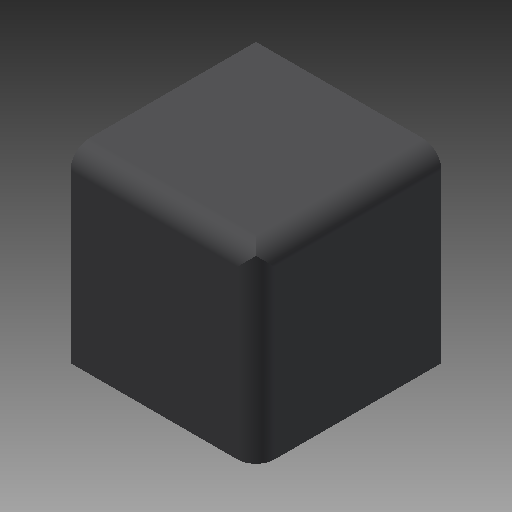
# Autodesk Inventor part: May Tec 1.48.14410_Corner piece set cubic PA
Saved by Autodesk Inventor 2018 (Build 220112000, 112)
## iProperties
Category: PARTsolutions
Company: MAYTEC
Created: 2012-11-13
Part Number: May Tec 1.48.14410_Corner piece set cubic PA
Catalog Web Link: www.cadenas.de
Description: 1.48.144xx-Corner pieces
Vendor: MAYTEC
Document SubType Name: Modeling
Designer: PARTuser1
Manufacturer: MAYTEC
Density: 1 g/cm^3
Material: Generic
Appearance: RGB(175.94999939203154,175.94999939203154,175.94999939203154)
PSOL_IDENT_0: {\\10.0.0.242\data_v9\23d-libs\maytec\maytec_3d\einbauzubehoer\eckstuecke\1.48.144xx.prj},234 {VTYP=
PSOL_IDENT_1: 3D},{NB=May Tec 1.48.14410_Corner piece set cubic PA},{LINA=May Tec 1.48.14410_Corner piece set cubi
PSOL_IDENT_2: c PA},{NN=1.48.144xx},{DATE=14.09.2010 08:34:28},{GEOMDATE=28.01.2010 00:00:00},{VERSION=},{LINEID=1
PSOL_IDENT_3: 0},{LINESUBID=-1},{WBVAR=}  {NB=May Tec 1.48.14410_Corner piece set cubic PA},{LINA=May Tec 1.48.144
PSOL_IDENT_4: 10_Corner piece set cubic PA},{KT=DUMMY},{PARTNR=1.48.14410},{DESCRIPTION=Eckstueck-Satz Quadrat PA}
PSOL_IDENT_5: ,{TYP=1},{XTRANS=Corner piece set cubic PA}
CNS_NT: Corner pieces
CNS_NB: May Tec 1.48.14410_Corner piece set cubic PA
CNS_NBSYN: May Tec $PARTNR._$XTRANS.
CNS_LINA: May Tec 1.48.14410_Corner piece set cubic PA
CNS_PARTNR: 1.48.14410
CNS_DESCRIPTION: Corner piece set cubic PA
CNS_TYP: 1
CNS_XTRANS: Corner piece set cubic PA
SUPPLIER: MAYTEC
ARTICLENO: May Tec 1.48.14410_Corner piece set cubic PA
BOMINFO: May Tec 1.48.14410_Corner piece set cubic PA
CREATOR: CADENAS GmbH
Title: May Tec 1.48.14410_Corner piece set cubic PA
Author: Cadenas PARTsolutions
Comments: Corner pieces
Autodesk Inventor part; units mm, degrees
sketch "Sketch_1" plane through (0, 0, 0) normal (0, 0, 1) x (1, 0, 0)
  line L0 (0, 0) -> (37, 0)
  line L1 (37, 0) -> (37, 5)
  line L2 (37, 5) -> (34.4991, 13.372)
  line L3 (34.4991, 13.372) -> (27.5772, 20.294)
  line L4 (27.5772, 20.294) -> (27.5772, 21.9203)
  line L5 (27.5772, 21.9203) -> (21.9203, 27.5772)
  line L6 (21.9203, 27.5772) -> (20.294, 27.5772)
  line L7 (20.294, 27.5772) -> (13.372, 34.4991)
  line L8 (13.372, 34.4991) -> (5, 37)
  line L9 (5, 37) -> (0, 37)
  line L10 (0, 37) -> (0, 0)
  circle A0 centre (19.852, 19.852) radius 4.425
  constraints: 22 end point, 1 centre point
extrude "Extrusion1" add sketch "Sketch_1" along normal blind 5
sketch "Sketch_2" plane through (0, 0, 0) normal (1, 0, 0) x (0, 1, 0)
  line L0 (0, 37) -> (0, 0)
  line L1 (0, 0) -> (37, 0)
  line L2 (37, 0) -> (37, 5)
  line L3 (37, 5) -> (34.4991, 13.372)
  line L4 (34.4991, 13.372) -> (27.5772, 20.294)
  line L5 (27.5772, 20.294) -> (27.5772, 21.9203)
  line L6 (27.5772, 21.9203) -> (21.9203, 27.5772)
  line L7 (21.9203, 27.5772) -> (20.294, 27.5772)
  line L8 (20.294, 27.5772) -> (13.372, 34.4991)
  line L9 (13.372, 34.4991) -> (5, 37)
  line L10 (5, 37) -> (0, 37)
  circle A0 centre (19.852, 19.852) radius 4.425
  constraints: 22 end point, 1 centre point
sketch "Sketch_3" plane through (0, 0, 0) normal (0, 1, 0) x (-1, 0, 0)
  line L0 (0, 37) -> (-5, 37)
  line L1 (-5, 37) -> (-13.372, 34.4991)
  line L2 (-13.372, 34.4991) -> (-20.294, 27.5772)
  line L3 (-20.294, 27.5772) -> (-21.9203, 27.5772)
  line L4 (-21.9203, 27.5772) -> (-27.5772, 21.9203)
  line L5 (-27.5772, 21.9203) -> (-27.5772, 20.294)
  line L6 (-27.5772, 20.294) -> (-34.4991, 13.372)
  line L7 (-34.4991, 13.372) -> (-37, 5)
  line L8 (-37, 5) -> (-37, 0)
  line L9 (-37, 0) -> (0, 0)
  line L10 (0, 0) -> (0, 37)
  circle A0 centre (-19.852, 19.852) radius 4.425
  constraints: 22 end point, 1 centre point
extrude "Extrusion2" add sketch "Sketch_3" along normal blind 5
extrude "Extrusion3" add sketch "Sketch_2" along normal blind 5
sketch "Sketch_4" plane through (0, 0, 0) normal (0, 0, 1) x (1, 0, 0)
  line L0 (2.5, 23.85) -> (2.5, 16.1)
  line L1 (2.5, 16.1) -> (4.35, 16.1)
  line L2 (4.35, 16.1) -> (4.35, 23.85)
  line L3 (4.35, 23.85) -> (2.5, 23.85)
  constraints: 8 end point
extrude "Extrusion4" add sketch "Sketch_4" against normal blind 4 draft -5
sketch "Sketch_5" plane through (0, 0, 0) normal (0, 0, 1) x (1, 0, 0)
  line L0 (16.1, 4.35) -> (16.1, 2.5)
  line L1 (16.1, 2.5) -> (23.85, 2.5)
  line L2 (23.85, 2.5) -> (23.85, 4.35)
  line L3 (23.85, 4.35) -> (16.1, 4.35)
  constraints: 8 end point
extrude "Extrusion5" add sketch "Sketch_5" against normal blind 4 draft -5
sketch "Sketch_6" plane through (0, 0, 0) normal (0, 0, 1) x (1, 0, 0)
  circle A0 centre (5.75, 12.975) radius 1
  constraints: 1 centre point
extrude "Extrusion6" add sketch "Sketch_6" against normal blind 4 draft -5
sketch "Sketch_7" plane through (0, 0, 0) normal (0, 0, 1) x (1, 0, 0)
  circle A0 centre (5.75, 26.975) radius 1
  constraints: 1 centre point
extrude "Extrusion7" add sketch "Sketch_7" against normal blind 4 draft -5
sketch "Sketch_8" plane through (0, 0, 0) normal (0, 0, 1) x (1, 0, 0)
  circle A0 centre (26.975, 5.75) radius 1
  constraints: 1 centre point
extrude "Extrusion8" add sketch "Sketch_8" against normal blind 4 draft -5
sketch "Sketch_9" plane through (0, 0, 0) normal (0, 0, 1) x (1, 0, 0)
  circle A0 centre (12.975, 5.75) radius 1
  constraints: 1 centre point
extrude "Extrusion9" add sketch "Sketch_9" against normal blind 4 draft -5
sketch "Sketch_10" plane through (0, 0, 0) normal (0, 1, 0) x (-1, 0, 0)
  line L0 (-2, 2) -> (-2, 8)
  line L1 (-2, 8) -> (-8, 8)
  line L2 (-8, 8) -> (-8, 2)
  line L3 (-8, 2) -> (-2, 2)
  constraints: 8 end point
extrude "Extrusion10" cut sketch "Sketch_10" along normal blind 8.5
sketch "Sketch_11" plane through (0, 0, 0) normal (0.7071068, 0, -0.7071068) x (-0.7071068, 0, -0.7071068)
  line L0 (-2, 0) -> (0, 0)
  line L1 (0, 0) -> (0, 2)
  line L2 (0, 2) -> (-2, 0)
  constraints: 6 end point
extrude "Extrusion11" cut sketch "Sketch_11" along normal mid plane 6
sketch "Sketch_12" plane through (0, 0, 0) normal (1, 0, 0) x (0, 1, 0)
  line L0 (23.85, 4.35) -> (16.1, 4.35)
  line L1 (16.1, 4.35) -> (16.1, 2.5)
  line L2 (16.1, 2.5) -> (23.85, 2.5)
  line L3 (23.85, 2.5) -> (23.85, 4.35)
  constraints: 8 end point
sketch "Sketch_13" plane through (0, 0, 0) normal (1, 0, 0) x (0, 1, 0)
  circle A0 centre (12.975, 5.75) radius 1
  constraints: 1 centre point
sketch "Sketch_14" plane through (0, 0, 0) normal (1, 0, 0) x (0, 1, 0)
  circle A0 centre (26.975, 5.75) radius 1
  constraints: 1 centre point
extrude "Extrusion12" add sketch "Sketch_14" against normal blind 4 draft -5
sketch "Sketch_15" plane through (0, 0, 0) normal (1, 0, 0) x (0, 1, 0)
  circle A0 centre (5.75, 12.975) radius 1
  constraints: 1 centre point
extrude "Extrusion13" add sketch "Sketch_15" against normal blind 4 draft -5
sketch "Sketch_16" plane through (0, 0, 0) normal (1, 0, 0) x (0, 1, 0)
  line L0 (4.35, 23.85) -> (2.5, 23.85)
  line L1 (2.5, 23.85) -> (2.5, 16.1)
  line L2 (2.5, 16.1) -> (4.35, 16.1)
  line L3 (4.35, 16.1) -> (4.35, 23.85)
  constraints: 8 end point
extrude "Extrusion14" add sketch "Sketch_16" against normal blind 4 draft -5
sketch "Sketch_17" plane through (0, 0, 0) normal (1, 0, 0) x (0, 1, 0)
  circle A0 centre (5.75, 26.975) radius 1
  constraints: 1 centre point
extrude "Extrusion15" add sketch "Sketch_17" against normal blind 4 draft -5
sketch "Sketch_18" plane through (0, 0, 0) normal (0, 1, 0) x (-1, 0, 0)
  line L0 (-16.1, 4.35) -> (-23.85, 4.35)
  line L1 (-23.85, 4.35) -> (-23.85, 2.5)
  line L2 (-23.85, 2.5) -> (-16.1, 2.5)
  line L3 (-16.1, 2.5) -> (-16.1, 4.35)
  constraints: 8 end point
extrude "Extrusion16" add sketch "Sketch_18" against normal blind 4 draft -5
sketch "Sketch_19" plane through (0, 0, 0) normal (0, 1, 0) x (-1, 0, 0)
  circle A0 centre (-12.975, 5.75) radius 1
  constraints: 1 centre point
extrude "Extrusion17" add sketch "Sketch_19" against normal blind 4 draft -5
sketch "Sketch_20" plane through (0, 0, 0) normal (0, 1, 0) x (-1, 0, 0)
  circle A0 centre (-26.975, 5.75) radius 1
  constraints: 1 centre point
extrude "Extrusion18" add sketch "Sketch_20" against normal blind 4 draft -5
sketch "Sketch_21" plane through (0, 0, 0) normal (0, 1, 0) x (-1, 0, 0)
  line L0 (-2.5, 23.85) -> (-4.35, 23.85)
  line L1 (-4.35, 23.85) -> (-4.35, 16.1)
  line L2 (-4.35, 16.1) -> (-2.5, 16.1)
  line L3 (-2.5, 16.1) -> (-2.5, 23.85)
  constraints: 8 end point
extrude "Extrusion19" add sketch "Sketch_21" against normal blind 4 draft -5
sketch "Sketch_22" plane through (0, 0, 0) normal (0, 1, 0) x (-1, 0, 0)
  circle A0 centre (-5.75, 12.975) radius 1
  constraints: 1 centre point
extrude "Extrusion20" add sketch "Sketch_22" against normal blind 4 draft -5
sketch "Sketch_23" plane through (0, 0, 0) normal (0, 1, 0) x (-1, 0, 0)
  circle A0 centre (-5.75, 26.975) radius 1
  constraints: 1 centre point
extrude "Extrusion21" add sketch "Sketch_23" against normal blind 4 draft -5
sketch "Sketch_24" plane through (0, 0, 0) normal (0, 0, 1) x (1, 0, 0)
  line L0 (0, 38) -> (36, 38)
  arc A0 (38, 36) -> (36, 38) centre (36, 36) ccw
  line L1 (38, 36) -> (38, 0)
  line L2 (38, 0) -> (40, 0)
  line L3 (40, 0) -> (40, 40)
  line L4 (40, 40) -> (0, 40)
  line L5 (0, 40) -> (0, 38)
  constraints: 12 end point, 2 point on circle, 1 centre point
sketch "Sketch_26" plane through (0, 0, 0) normal (0.7071068, 0, -0.7071068) x (-0.7071068, 0, -0.7071068)
  line L0 (-7.3236, 5.2311) -> (-51.8655, 37.0468)
  line L1 (-51.8655, 37.0468) -> (-50.3543, 39.1625)
  line L2 (-50.3543, 39.1625) -> (-5.8124, 7.3469)
  line L3 (-5.8124, 7.3469) -> (-7.3236, 5.2311)
  line L4 (-7.3236, 5.2311) -> (-51.8655, 37.0468)
  constraints: 10 end point
revolve "Revolution1" add sketch "Sketch_26" angle 360 about axis through (5.1786, 5.2311, 5.1786) along (-0.5753965, -0.5812382, -0.5753965)
extrude "Extrusion22" add sketch "Sketch_24" along normal blind 40
sketch "Sketch_28" plane through (0, 0, 0) normal (1, 0, 0) x (0, 1, 0)
  line L0 (42, 42) -> (36, 42)
  line L1 (36, 42) -> (36, 40)
  arc A0 (40, 36) -> (36, 40) centre (36, 36) ccw
  line L2 (40, 36) -> (42, 36)
  line L3 (42, 36) -> (42, 42)
  constraints: 8 end point, 2 point on circle, 1 centre point
extrude "Extrusion23" cut sketch "Sketch_28" along normal blind 40
sketch "Sketch_29" plane through (0, 0, 0) normal (1, 0, 0) x (0, 1, 0)
  line L0 (0, 40) -> (0, 38)
  line L1 (0, 38) -> (36, 38)
  arc A0 (38, 36) -> (36, 38) centre (36, 36) ccw
  line L2 (38, 36) -> (38, 0)
  line L3 (38, 0) -> (40, 0)
  line L4 (40, 0) -> (40, 40)
  line L5 (40, 40) -> (0, 40)
  constraints: 12 end point, 2 point on circle, 1 centre point
extrude "Extrusion24" add sketch "Sketch_29" along normal blind 40
sketch "Sketch_25" plane through (0, 0, 0) normal (1, 0, 0) x (0, 1, 0)
  arc A0 (40, 36) -> (36, 40) centre (36, 36) ccw
  line L0 (40, 36) -> (40, 40)
  line L1 (40, 40) -> (36, 40)
  constraints: 4 end point, 2 point on circle, 1 centre point
extrude "Extrusion25" cut sketch "Sketch_25" along normal blind 40
sketch "Sketch_27" plane through (0, 0, 0) normal (0, 0, 1) x (1, 0, 0)
  arc A0 (40, 36) -> (36, 40) centre (36, 36) ccw
  line L0 (40, 36) -> (40, 40)
  line L1 (40, 40) -> (36, 40)
  constraints: 4 end point, 2 point on circle, 1 centre point
extrude "Extrusion26" cut sketch "Sketch_27" along normal blind 40
sketch "Sketch_30" plane through (0, 0, 0) normal (0, 1, 0) x (-1, 0, 0)
  line L0 (-36, 40) -> (-40, 40)
  line L1 (-40, 40) -> (-40, 36)
  arc A0 (-36, 40) -> (-40, 36) centre (-36, 36) ccw
  constraints: 4 end point, 2 point on circle, 1 centre point
sketch "Sketch_31" plane through (0, 0, 0) normal (0, 1, 0) x (-1, 0, 0)
  line L0 (-36, 38) -> (-36, 40)
  arc A0 (-36, 40) -> (-40, 36) centre (-36, 36) ccw
  line L1 (-40, 36) -> (-38, 36)
  arc A1 (-36, 38) -> (-38, 36) centre (-36, 36) ccw
  constraints: 4 end point, 4 point on circle, 2 centre point
extrude "Extrusion27" add sketch "Sketch_31" along normal blind 36
extrude "Extrusion28" cut sketch "Sketch_30" along normal blind 40
extrude "Extrusion29" add sketch "Sketch_12" against normal blind 4 draft -5
extrude "Extrusion30" add sketch "Sketch_13" against normal blind 4 draft -5
ref_plane "side_1_XY" through (19.852, 19.852, 0) normal (0, 0, -1) x (1, 0, 0)
ref_plane "side_1_YZ" through (19.852, 19.852, 0) normal (1, 0, 0) x (0, -1, 0)
ref_plane "side_1_ZX" through (19.852, 19.852, 0) normal (0, -1, 0) x (0, 0, -1)
ref_plane "side_2_XY" through (19.852, 0, 19.852) normal (0, -1, 0) x (1, 0, 0)
ref_plane "side_2_YZ" through (19.852, 0, 19.852) normal (1, 0, 0) x (0, 0, 1)
ref_plane "side_2_ZX" through (19.852, 0, 19.852) normal (0, 0, 1) x (0, -1, 0)
ref_plane "side_3_XY" through (0, 19.852, 19.852) normal (-1, 0, 0) x (0, 0, -1)
ref_plane "side_3_YZ" through (0, 19.852, 19.852) normal (0, 0, -1) x (0, -1, 0)
ref_plane "side_3_ZX" through (0, 19.852, 19.852) normal (0, -1, 0) x (-1, 0, 0)
body "Solid1"
